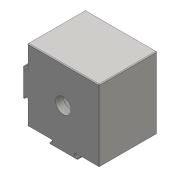
# Autodesk Inventor part: Tool Post
Saved by Autodesk Inventor 2016 (Build 200138000, 138)
## iProperties
Created: 2020-10-21
Part Number: Tool Post
Material: Generic
Document SubType Name: Modeling
Designer: extract
Density: 1 g/cm^3
Appearance: Default
Author: extract
Autodesk Inventor part; units mm, degrees
ref_plane "YZ Plane" through (0, 0, 0) normal (1, 0, 0) x (0, 1, 0)
ref_plane "XZ Plane" through (0, 0, 0) normal (0, 1, 0) x (-1, 0, 0)
ref_plane "XY Plane" through (0, 0, 0) normal (0, 0, 1) x (1, 0, 0)
sketch "Sketch1" plane through (0, 0, 0) normal (0, 1, 0) x (-1, 0, 0)
  line L0 (-23.5, 23.5) -> (23.5, 23.5)
  line L1 (26.5, 10) -> (26.5, -10)
  line L2 (10, -26.5) -> (-10, -26.5)
  line L3 (-23.5, -23.5) -> (-23.5, 23.5)
  line L4 (26.5, 10) -> (23.5, 7)
  line L5 (23.5, 7) -> (23.5, 23.5)
  line L6 (26.5, -10) -> (23.5, -7)
  line L7 (23.5, -7) -> (23.5, -23.5)
  line L8 (23.5, -23.5) -> (7, -23.5)
  line L9 (7, -23.5) -> (10, -26.5)
  line L10 (-23.5, -23.5) -> (-7, -23.5)
  line L11 (-7, -23.5) -> (-10, -26.5)
  line L12 (0, 0) -> (0, -23.5) construction
  line L13 (0, 0) -> (0, 23.5) construction
  line L14 (0, 0) -> (23.5, 0) construction
  line L15 (0, 0) -> (-23.5, 0) construction
  line L16 (7, -23.5) -> (-7, -23.5) construction
  line L17 (23.5, 7) -> (23.5, -7) construction
  line L18 (23.5, 23.5) -> (-23.5, -23.5) construction
  line L19 (23.5, -23.5) -> (-23.5, 23.5) construction
  dimension "d2" = 45
  dimension "d3" = 45
  dimension "d4" = 3
  dimension "d5" = 45
  dimension "d6" = 45
  dimension "d13" = 50
  dimension "d14" = 50
  dimension "d16" = 20
  constraints: 40 end point, 6 equal length, 5 horizontal, 4 midpoint, 3 collinear, 3 perpendicular, 2 parallel, 2 vertical, 1 coincident, 1 point on line
  measures "d2" angle of L7 L6
  measures "d3" angle of L5 L4
  measures "d4" distance between parallel lines of L5 L1
  measures "d5" angle of L11 L10
  measures "d6" angle of L9 L8
  measures "d13" distance between parallel lines of L2 L0
  measures "d14" distance between parallel lines of L3 L1
  measures "d16" distance of L1.start L1.end
extrude "Extrusion1" add sketch "Sketch1" along normal blind 38
fillet "Fillet1" radius 0.5 36 edges at (0, 0, 23.5) (-23.5, 0, 15.25) (-25, 0, 8.5) (-26.5, 0, 0) (-25, 0, -8.5) (-23.5, 0, -15.25) (-15.25, 0, -23.5) (-8.5, 0, -25) (0, 0, -26.5) (8.5, 0, -25) (15.25, 0, -23.5) (23.5, 0, 0) (0, 38, 23.5) (23.5, 38, 0) (15.25, 38, -23.5) (8.5, 38, -25) (0, 38, -26.5) (-8.5, 38, -25) (-15.25, 38, -23.5) (-23.5, 38, -15.25) (-25, 38, -8.5) (-26.5, 38, 0) (-25, 38, 8.5) (-23.5, 38, 15.25) (-23.5, 19, 23.5) (-23.5, 19, 7) (-26.5, 19, 10) (-26.5, 19, -10) (-23.5, 19, -7) (-23.5, 19, -23.5) (-7, 19, -23.5) (-10, 19, -26.5) (10, 19, -26.5) (7, 19, -23.5) (23.5, 19, -23.5) (23.5, 19, 23.5)
sketch "Sketch2" plane through (0, 38, 0) normal (0, 1, 0) x (1, 0, 0)
  circle A0 centre (0, 0) radius 10
  dimension "d17" = 20
  constraints: 1 centre point, 1 coincident
  measures "d17" diameter of A0
extrude "Extrusion2" cut sketch "Sketch2" against normal blind 33
sketch "Sketch3" plane through (0, 5, 0) normal (0, 1, 0) x (1, 0, 0)
  circle A0 centre (0, 0) radius 5
  dimension "d20" = 10
  constraints: 1 centre point, 1 coincident
  measures "d20" diameter of A0
extrude "Extrusion3" cut sketch "Sketch3" against normal through all
chamfer "Chamfer2" distance 1 angle 45 1 edges at (-10, 38, 0)
body "Solid1"
